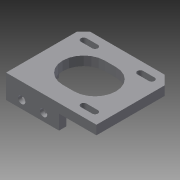
# Autodesk Inventor part: Y motor mount
Saved by Autodesk Inventor 2014 SP1 (Build 180222100, 222)
## iProperties
Created: 2015-07-22
Part Number: Y motor mount
Material: Generic
Document SubType Name: Modeling
Designer: Mon
Density: 1 g/cm^3
Appearance: Default
Author: Mon
Autodesk Inventor part; units mm, degrees
ref_plane "YZ Plane" through (0, 0, 0) normal (1, 0, 0) x (0, 1, 0)
ref_plane "XZ Plane" through (0, 0, 0) normal (0, 1, 0) x (-1, 0, 0)
ref_plane "XY Plane" through (0, 0, 0) normal (0, 0, 1) x (1, 0, 0)
sketch "Sketch2" plane through (0, 0, 0) normal (0, 0, 1) x (1, 0, 0)
  line L0 (49.4803, 37.44) -> (44.4803, 42.44)
  line L1 (5.7803, 38.32) -> (5.3662, 38.2655)
  line L2 (4.9803, 38.1056) -> (4.6489, 37.8514)
  line L3 (3.4803, 42.44) -> (44.4803, 42.44)
  line L4 (-0.0197, 38.94) -> (3.4803, 42.44)
  line L5 (-0.0197, 0) -> (49.4803, 0)
  line L6 (49.4803, 37.44) -> (49.4803, 0)
  line L7 (4.2348, 36.3059) -> (4.3946, 35.92)
  line L8 (10.1721, 18.2436) -> (11.321, 15.47)
  line L9 (35.2348, 6.1341) -> (35.1803, 5.72)
  line L10 (4.6489, 35.5886) -> (4.9803, 35.3344)
  line L11 (36.7803, 38.32) -> (36.3662, 38.2655)
  line L12 (36.3662, 35.1745) -> (36.7803, 35.12)
  line L13 (35.3946, 35.92) -> (35.6489, 35.5886)
  line L14 (35.1803, 36.72) -> (35.2348, 36.3059)
  line L15 (35.2348, 5.3059) -> (35.3946, 4.92)
  line L16 (21.2803, 32.72) -> (18.3039, 32.3281)
  line L17 (35.2348, 37.1341) -> (35.1803, 36.72)
  line L18 (35.3946, 6.52) -> (35.2348, 6.1341)
  line L19 (35.9803, 7.1056) -> (35.6489, 6.8514)
  line L20 (36.7803, 7.32) -> (36.3662, 7.2655)
  line L21 (35.6489, 6.8514) -> (35.3946, 6.52)
  line L22 (35.9803, 35.3344) -> (36.3662, 35.1745)
  line L23 (4.6489, 37.8514) -> (4.3946, 37.52)
  line L24 (5.3662, 38.2655) -> (4.9803, 38.1056)
  line L25 (4.3946, 35.92) -> (4.6489, 35.5886)
  line L26 (35.6489, 35.5886) -> (35.9803, 35.3344)
  line L27 (36.3662, 38.2655) -> (35.9803, 38.1056)
  line L28 (5.3662, 35.1745) -> (5.7803, 35.12)
  line L29 (4.9803, 35.3344) -> (5.3662, 35.1745)
  line L30 (4.1803, 36.72) -> (4.2348, 36.3059)
  line L31 (4.2348, 37.1341) -> (4.1803, 36.72)
  line L32 (4.3946, 37.52) -> (4.2348, 37.1341)
  line L33 (18.3039, 10.1119) -> (21.2803, 9.72)
  line L34 (15.5303, 11.2607) -> (18.3039, 10.1119)
  line L35 (13.1485, 13.0883) -> (15.5303, 11.2607)
  line L36 (11.321, 15.47) -> (13.1485, 13.0883)
  line L37 (9.7803, 21.22) -> (10.1721, 18.2436)
  line L38 (10.1721, 24.1964) -> (9.7803, 21.22)
  line L39 (11.321, 26.97) -> (10.1721, 24.1964)
  line L40 (13.1485, 29.3517) -> (11.321, 26.97)
  line L41 (15.5303, 31.1793) -> (13.1485, 29.3517)
  line L42 (18.3039, 32.3281) -> (15.5303, 31.1793)
  line L43 (36.3662, 7.2655) -> (35.9803, 7.1056)
  line L44 (36.3662, 4.1745) -> (36.7803, 4.12)
  line L45 (35.9803, 4.3344) -> (36.3662, 4.1745)
  line L46 (35.6489, 4.5886) -> (35.9803, 4.3344)
  line L47 (35.3946, 4.92) -> (35.6489, 4.5886)
  line L48 (35.1803, 5.72) -> (35.2348, 5.3059)
  line L49 (35.2348, 36.3059) -> (35.3946, 35.92)
  line L50 (35.3946, 37.52) -> (35.2348, 37.1341)
  line L51 (35.6489, 37.8514) -> (35.3946, 37.52)
  line L52 (35.9803, 38.1056) -> (35.6489, 37.8514)
  line L53 (27.4803, 9.72) -> (30.4567, 10.1119)
  line L54 (35.612, 29.3517) -> (33.2303, 31.1793)
  line L55 (38.5884, 24.1964) -> (37.4396, 26.97)
  line L56 (12.7803, 35.3344) -> (13.1116, 35.5886)
  line L57 (30.4567, 10.1119) -> (33.2303, 11.2607)
  line L58 (38.9803, 21.22) -> (38.5884, 24.1964)
  line L59 (43.7803, 35.3344) -> (44.1116, 35.5886)
  line L60 (44.5257, 6.1341) -> (44.3659, 6.52)
  line L61 (38.5884, 18.2436) -> (38.9803, 21.22)
  line L62 (44.3659, 37.52) -> (44.1116, 37.8514)
  line L63 (44.1116, 37.8514) -> (43.7803, 38.1056)
  line L64 (13.3659, 35.92) -> (13.5258, 36.3059)
  line L65 (44.1116, 4.5886) -> (44.3659, 4.92)
  line L66 (43.3944, 38.2655) -> (42.9803, 38.32)
  line L67 (30.4567, 32.3281) -> (27.4803, 32.72)
  line L68 (44.1116, 35.5886) -> (44.3659, 35.92)
  line L69 (35.612, 13.0883) -> (37.4396, 15.47)
  line L70 (37.4396, 26.97) -> (35.612, 29.3517)
  line L71 (37.4396, 15.47) -> (38.5884, 18.2436)
  line L72 (43.7803, 4.3344) -> (44.1116, 4.5886)
  line L73 (13.1116, 37.8514) -> (12.7803, 38.1056)
  line L74 (33.2303, 31.1793) -> (30.4567, 32.3281)
  line L75 (12.7803, 38.1056) -> (12.3944, 38.2655)
  line L76 (44.3659, 6.52) -> (44.1116, 6.8514)
  line L77 (33.2303, 11.2607) -> (35.612, 13.0883)
  line L78 (42.9803, 4.12) -> (43.3944, 4.1745)
  line L79 (44.5257, 37.1341) -> (44.3659, 37.52)
  line L80 (43.7803, 7.1056) -> (43.3944, 7.2655)
  line L81 (44.5257, 5.3059) -> (44.5803, 5.72)
  line L82 (43.7803, 38.1056) -> (43.3944, 38.2655)
  line L83 (12.3944, 38.2655) -> (11.9803, 38.32)
  line L84 (44.3659, 35.92) -> (44.5257, 36.3059)
  line L85 (43.3944, 35.1745) -> (43.7803, 35.3344)
  line L86 (43.3944, 4.1745) -> (43.7803, 4.3344)
  line L87 (13.1116, 35.5886) -> (13.3659, 35.92)
  line L88 (11.9803, 35.12) -> (12.3944, 35.1745)
  line L89 (42.9803, 35.12) -> (43.3944, 35.1745)
  line L90 (44.5803, 5.72) -> (44.5257, 6.1341)
  line L91 (43.3944, 7.2655) -> (42.9803, 7.32)
  line L92 (13.5258, 36.3059) -> (13.5803, 36.72)
  line L93 (44.3659, 4.92) -> (44.5257, 5.3059)
  line L94 (13.5258, 37.1341) -> (13.3659, 37.52)
  line L95 (44.5803, 36.72) -> (44.5257, 37.1341)
  line L96 (44.5257, 36.3059) -> (44.5803, 36.72)
  line L97 (13.3659, 37.52) -> (13.1116, 37.8514)
  line L98 (44.1116, 6.8514) -> (43.7803, 7.1056)
  line L99 (12.3944, 35.1745) -> (12.7803, 35.3344)
  line L100 (13.5803, 36.72) -> (13.5258, 37.1341)
  line L101 (5.7803, 38.32) -> (11.9803, 38.32)
  line L102 (5.7803, 35.12) -> (11.9803, 35.12)
  line L103 (36.7803, 35.12) -> (42.9803, 35.12)
  line L104 (36.7803, 7.32) -> (42.9803, 7.32)
  line L105 (36.7803, 4.12) -> (42.9803, 4.12)
  line L106 (21.2803, 32.72) -> (27.4803, 32.72)
  line L107 (21.2803, 9.72) -> (27.4803, 9.72)
  line L108 (36.7803, 38.32) -> (42.9803, 38.32)
  line L109 (-0.0197, 0) -> (-0.0197, 38.94)
  point P0 (0, 0)
  constraints: 220 end point
extrude "Extrusion1" add sketch "Sketch2" along normal blind 5
sketch "Sketch3" plane through (0, 0, 0) normal (0, 0, -1) x (-1, 0, 0)
  line L0 (0, 0) -> (-4, 0)
  line L1 (-4, 0) -> (-4, 25)
  line L2 (-4, 25) -> (0, 25)
  line L3 (0, 25) -> (0, 0)
  dimension "d2" = 4
  dimension "d3" = 25
  constraints: 8 end point, 2 parallel, 1 horizontal, 1 perpendicular
  measures "d2" distance of L1.end L2.end
  measures "d3" distance of L0.end L1.end
extrude "Extrusion2" add sketch "Sketch3" along normal blind 8
sketch "Sketch4" plane through (0, 0, 0) normal (0, 0, -1) x (-1, 0, 0)
  line L0 (-4, 0) -> (-29, 0)
  line L1 (-29, 0) -> (-29, 4)
  line L2 (-29, 4) -> (-4, 4)
  line L3 (-4, 4) -> (-4, 0)
  dimension "d6" = 25
  dimension "d7" = 4
  constraints: 8 end point, 2 parallel, 1 horizontal, 1 perpendicular
  measures "d6" distance of L1.end L2.end
  measures "d7" distance of L0.end L1.end
extrude "Extrusion3" add sketch "Sketch4" along normal blind 8
sketch "Sketch5" plane through (0, 0, 0) normal (-1, 0, 0) x (0, 0, 1)
  line L0 (0, 25) -> (0, 0) projected
  line L1 (0, 25) -> (-8, 25) projected
  line L2 (-8, 0) -> (-8, 25) projected
  line L3 (0, 0) -> (-8, 0) projected
  line L4 (-12.7767, 12.5) -> (11.2598, 12.5)
  line L5 (-4, 28.2185) -> (-4, -2.7903)
  constraints: 4 end point, 1 parallel, 1 perpendicular
hole "Hole1" at (0, 7.828, -4) direction (1, 0, 0) diameter 4 end through all
hole "Hole2" at (0, 18.6411, -4.0217) direction (1, 0, 0) diameter 4 end through all
hole "Hole3" at (20.5377, 0, -3.7583) direction (0, 1, 0) diameter 4 end through all
hole "Hole4" at (8.5455, 0, -3.6478) direction (0, 1, 0) diameter 4 end through all
sketch "Sketch8" plane through (4, 25, 0) normal (1, 0, 0) x (0, 0, -1)
  circle A0 centre (4.0217, -6.3589) radius 2 projected
  line L0 (3.7794, -9.5251) -> (1.1586, -7.7322)
  line L1 (1.1586, -7.7322) -> (1.4009, -4.566)
  line L2 (1.4009, -4.566) -> (4.264, -3.1927)
  line L3 (4.264, -3.1927) -> (6.8849, -4.9857)
  line L4 (6.8849, -4.9857) -> (6.6425, -8.1518)
  line L5 (6.6425, -8.1518) -> (3.7794, -9.5251)
  point P0 (0, -25)
  point P1 (5.211, -8.8385)
  constraints: 12 end point, 1 midpoint, 13 other
extrude "Extrusion6" cut sketch "Sketch8" against normal blind 2
sketch "Sketch11" plane through (4, 25, 0) normal (1, 0, 0) x (0, 0, -1)
  circle A0 centre (4, -17.172) radius 2 projected
  line L0 (6.75, -18.7597) -> (4, -20.3474)
  line L1 (4, -20.3474) -> (1.25, -18.7597)
  line L2 (1.25, -18.7597) -> (1.25, -15.5843)
  line L3 (1.25, -15.5843) -> (4, -13.9966)
  line L4 (4, -13.9966) -> (6.75, -15.5843)
  line L5 (6.75, -15.5843) -> (6.75, -18.7597)
  point P0 (0, -25)
  point P1 (6.75, -17.172)
  constraints: 12 end point, 1 midpoint, 13 other
extrude "Extrusion8" cut sketch "Sketch11" against normal blind 2
sketch "Sketch12" plane through (4, 4, 0) normal (0, 1, 0) x (1, 0, 0)
  circle A0 centre (4.5455, 3.6478) radius 2 projected
  line L0 (7.2955, 2.0601) -> (4.5455, 0.4724)
  line L1 (4.5455, 0.4724) -> (1.7955, 2.0601)
  line L2 (1.7955, 2.0601) -> (1.7955, 5.2355)
  line L3 (1.7955, 5.2355) -> (4.5455, 6.8232)
  line L4 (4.5455, 6.8232) -> (7.2954, 5.2355)
  line L5 (7.2954, 5.2355) -> (7.2955, 2.0601)
  point P0 (-4, 0)
  point P1 (7.2955, 3.6478)
  constraints: 12 end point, 1 midpoint, 13 other
extrude "Extrusion9" cut sketch "Sketch12" against normal blind 2
sketch "Sketch13" plane through (4, 4, 0) normal (0, 1, 0) x (1, 0, 0)
  circle A0 centre (16.5377, 3.7583) radius 2 projected
  line L0 (18.143, 1.0186) -> (14.9677, 0.9981)
  line L1 (14.9677, 0.9981) -> (13.3623, 3.7379)
  line L2 (13.3623, 3.7379) -> (14.9323, 6.498)
  line L3 (14.9323, 6.498) -> (18.1076, 6.5185)
  line L4 (18.1076, 6.5185) -> (19.713, 3.7788)
  line L5 (19.713, 3.7788) -> (18.143, 1.0186)
  point P0 (-4, 0)
  point P1 (18.928, 2.3987)
  constraints: 12 end point, 1 midpoint, 13 other
extrude "Extrusion10" cut sketch "Sketch13" against normal blind 2
body "Solid1"
